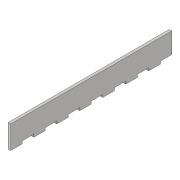
# Autodesk Inventor part: wall
Saved by Autodesk Inventor 2017 (Build 210142000, 142)
## iProperties
Created: 2019-06-11
Part Number: wall
Material: Generic
Document SubType Name: Modeling
Designer: markg
Density: 1 g/cm^3
Appearance: Default
Author: markg
Autodesk Inventor part; units mm, degrees
ref_plane "YZ Plane" through (0, 0, 0) normal (1, 0, 0) x (0, 1, 0)
ref_plane "XZ Plane" through (0, 0, 0) normal (0, 1, 0) x (-1, 0, 0)
ref_plane "XY Plane" through (0, 0, 0) normal (0, 0, 1) x (1, 0, 0)
sketch "Sketch1" plane through (0, 0, 0) normal (1, 0, 0) x (0, 1, 0)
  line L0 (0, 80.3974) -> (25.4, 80.3974)
  line L1 (25.4, 80.3974) -> (25.4, -97.4026)
  line L2 (25.4, -97.4026) -> (0, -97.4026)
  line L3 (0, -97.4026) -> (0, 80.3974)
  point P0 (0, 0)
  dimension "d0" = 177.8
  dimension "d1" = 25.4
  dimension "d2" = 0
  constraints: 8 end point, 2 parallel, 1 horizontal, 1 perpendicular
  measures "d0" distance of L0.end L1.end
  measures "d1" distance of L0.start L0.end
  measures "d2" distance from line of L3 point (0, 0)
extrude "Extrusion1" add sketch "Sketch1" along normal blind 2.921
sketch "Sketch2" plane through (2.921, 0, 0) normal (1, 0, 0) x (0, 0, -1)
  line L0 (-80.3974, 0) -> (97.4026, 0) projected
  line L1 (-67.6974, 0) -> (-54.9974, 0)
  line L2 (-54.9974, 0) -> (-54.9974, 2.921)
  line L3 (-54.9974, 2.921) -> (-67.6974, 2.921)
  line L4 (-67.6974, 2.921) -> (-67.6974, 0)
  line L5 (-80.3974, 25.4) -> (-80.3974, 0) projected
  line L6 (-42.2974, 0) -> (-29.5974, 0)
  line L7 (-29.5974, 0) -> (-29.5974, 2.921)
  line L8 (-29.5974, 2.921) -> (-42.2974, 2.921)
  line L9 (-42.2974, 2.921) -> (-42.2974, 0)
  line L10 (-16.8974, 0) -> (-4.1974, 0)
  line L11 (-4.1974, 0) -> (-4.1974, 2.921)
  line L12 (-4.1974, 2.921) -> (-16.8974, 2.921)
  line L13 (-16.8974, 2.921) -> (-16.8974, 0)
  line L14 (8.5026, 0) -> (21.2026, 0)
  line L15 (21.2026, 0) -> (21.2026, 2.921)
  line L16 (21.2026, 2.921) -> (8.5026, 2.921)
  line L17 (8.5026, 2.921) -> (8.5026, 0)
  line L18 (33.9026, 0) -> (46.6026, 0)
  line L19 (46.6026, 0) -> (46.6026, 2.921)
  line L20 (46.6026, 2.921) -> (33.9026, 2.921)
  line L21 (33.9026, 2.921) -> (33.9026, 0)
  line L22 (59.3026, 0) -> (72.0026, 0)
  line L23 (72.0026, 0) -> (72.0026, 2.921)
  line L24 (72.0026, 2.921) -> (59.3026, 2.921)
  line L25 (59.3026, 2.921) -> (59.3026, 0)
  line L26 (84.7026, 0) -> (97.4026, 0)
  line L27 (97.4026, 0) -> (97.4026, 2.921)
  line L28 (97.4026, 2.921) -> (84.7026, 2.921)
  line L29 (84.7026, 2.921) -> (84.7026, 0)
  point P0 (0, 0)
  dimension "d5" = 12.7
  dimension "d6" = 2.921
  dimension "d7" = 12.7
  dimension "d10" = 25.4
  constraints: 56 end point, 2 horizontal, 2 parallel, 1 collinear, 1 perpendicular, 1 point on line, 47 other
  measures "d5" distance of L2.end L3.end
  measures "d6" distance of L3.end L1.start
  measures "d7" distance between parallel lines of L4 L5
  measures "d10" distance of L1.start L6.start
extrude "Extrusion2" cut sketch "Sketch2" against normal blind 2.921
body "Solid1"
